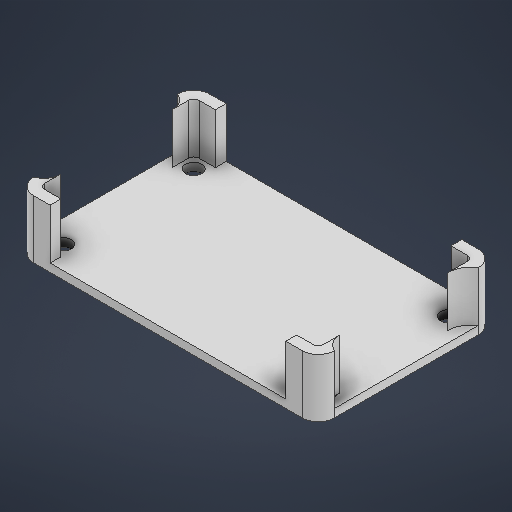
# Autodesk Inventor part: Part4
Saved by Autodesk Inventor 2026.1 (Build 301233020, 233B)
## iProperties
Created: 2025-12-24
Part Number: Part4
Material: Generic
Document SubType Name: Modeling
Designer: ferrm
Density: 1 g/cm^3
Appearance: Default
Author: ferrm
Autodesk Inventor part; units mm, degrees
ref_plane "YZ Plane" through (0, 0, 0) normal (1, 0, 0) x (0, 1, 0)
ref_plane "XZ Plane" through (0, 0, 0) normal (0, 1, 0) x (-1, 0, 0)
ref_plane "XY Plane" through (0, 0, 0) normal (0, 0, 1) x (1, 0, 0)
sketch "Sketch3" plane through (0, 0, 0) normal (0, 1, 0) x (-1, 0, 0)
  line L0 (-25.75, 13.25) -> (-25.75, -13.25)
  line L1 (-24.75, -14.25) -> (24.75, -14.25)
  line L2 (25.75, -13.25) -> (25.75, 13.25)
  line L3 (24.75, 14.25) -> (-24.75, 14.25)
  arc A0 (-25.75, -13.25) -> (-24.75, -14.25) centre (-24.75, -13.25) ccw
  arc A1 (-24.75, 14.25) -> (-25.75, 13.25) centre (-24.75, 13.25) ccw
  arc A2 (25.75, 13.25) -> (24.75, 14.25) centre (24.75, 13.25) ccw
  arc A3 (24.75, -14.25) -> (25.75, -13.25) centre (24.75, -13.25) ccw
  line L4 (24.75, -16.25) -> (-24.75, -16.25)
  arc A4 (-27.75, -13.25) -> (-24.75, -16.25) centre (-24.75, -13.25) ccw
  line L5 (-27.75, -13.25) -> (-27.75, 13.25)
  arc A5 (-24.75, 16.25) -> (-27.75, 13.25) centre (-24.75, 13.25) ccw
  line L6 (-24.75, 16.25) -> (24.75, 16.25)
  arc A6 (27.75, 13.25) -> (24.75, 16.25) centre (24.75, 13.25) ccw
  line L7 (27.75, 13.25) -> (27.75, -13.25)
  arc A7 (24.75, -16.25) -> (27.75, -13.25) centre (24.75, -13.25) ccw
  line L8 (21.75, -16.25) -> (21.75, -14.25)
  line L9 (27.75, -10.25) -> (25.75, -10.25)
  line L10 (25.75, 10.25) -> (27.75, 10.25)
  line L11 (21.75, 14.25) -> (21.75, 16.25)
  line L12 (-21.75, 14.25) -> (-21.75, 16.25)
  line L13 (-25.75, 10.25) -> (-27.75, 10.25)
  line L14 (-25.75, -10.25) -> (-27.75, -10.25)
  line L15 (-21.75, -16.25) -> (-21.75, -14.25)
  line L16 (-21.75, -14.25) -> (-17.75, -14.25)
  arc A8 (-17.75, -14.25) -> (-21.75, -16.25) centre (-15.3911, -23.9678) ccw
  line L17 (-21.75, 14.25) -> (-17.75, 14.25)
  arc A9 (-21.75, 16.25) -> (-17.75, 14.25) centre (-15.3911, 23.9678) ccw
  line L18 (-25.75, -10.25) -> (-25.75, -6.2495)
  line L19 (-25.75, 10.25) -> (-25.75, 6.25)
  arc A10 (-27.75, -10.25) -> (-25.75, -6.2495) centre (-35.468, -3.8913) ccw
  arc A11 (-25.75, 6.25) -> (-27.75, 10.25) centre (-35.4678, 3.8911) ccw
  line L20 (25.75, -10.25) -> (25.75, -6.2495)
  arc A12 (25.75, -6.2495) -> (27.75, -10.25) centre (35.468, -3.8913) ccw
  line L21 (25.75, 10.25) -> (25.75, 6.25)
  arc A13 (27.75, 10.25) -> (25.75, 6.25) centre (35.4678, 3.8911) ccw
  point P0 (0, 0)
  point P1 (0, 0)
  point P2 (-25.75, 14.25)
  point P3 (-25.75, -14.25)
  point P4 (25.75, -14.25)
  point P5 (21.75, 15.25)
  point P6 (-26.75, 10.25)
  dimension "d8" = 28.5
  dimension "d9" = 51.5
  dimension "d10" = 14.25
  dimension "d11" = 25.75
  dimension "d12" = 1
  dimension "d13" = 2
  dimension "d14" = 3
  dimension "d15" = 3
  dimension "d16" = 3
  dimension "d17" = 3
  dimension "d18" = 3
  dimension "d19" = 3
  dimension "d20" = 3
  dimension "d21" = 3
  dimension "d22" = 4
  dimension "d23" = 10
  dimension "d24" = 10
  dimension "d25" = 4
  dimension "d26" = 10
  dimension "d27" = 10
  dimension "d28" = 10
  dimension "d29" = 10
  constraints: 44 end point, 28 point on circle, 28 point on line, 14 centre point, 11 perpendicular, 8 tangent, 3 equal radius, 2 horizontal, 2 midpoint, 1 coincident, 1 vertical, 7 other
  measures "d8" distance of point (-25.75, 14.25) point (-25.75, -14.25)
  measures "d9" distance of point (-25.75, -14.25) point (25.75, -14.25)
  measures "d10" vertical distance of point (0, 0) point (-25.75, -14.25)
  measures "d11" horizontal distance of point (0, 0) point (-25.75, -14.25)
  measures "d12" radius of A0
  measures "d13" distance between parallel lines of L1 L4
  measures "d14" distance of L4.start L8.start
  measures "d15" distance from line of L7.end L9
  measures "d16" distance of L7.start L10.end
  measures "d17" horizontal distance of L6.end point (21.75, 15.25)
  measures "d18" distance of L6.start L12.end
  measures "d19" vertical distance of L5.end point (-26.75, 10.25)
  measures "d20" distance from line of L0.end L14
  measures "d21" distance of L15.start L4.end
  measures "d22" distance of L16.start L16.end
  measures "d23" radius of A8
  measures "d24" radius of A9
  measures "d25" distance of L13.start L19.end
  measures "d26" radius of A10
  measures "d27" radius of A11
  measures "d28" radius of A12
  measures "d29" radius of A13
extrude "Extrusion2" add sketch "Sketch3" along normal blind 3 contours L0 L13 L5 A5 L6 L12 L3 A1 | L0 A11 L13 | L12 A9 L3 | L0 L14 A10 | L14 L0 A0 L1 L15 L4 A4 L5 | L11 L6 A6 L7 L10 L2 A2 L3 | L15 L1 A8 | L8 L1 A3 L2 L9 L7 A7 L4 | L10 A13 L2 | L9 L2 A12
sketch "Sketch4" plane through (0, 0, 0) normal (0, -1, 0) x (1, 0, 0)
  line L0 (-27.75, -13.25) -> (-27.75, -10.25) projected
  arc A0 (-27.75, -13.25) -> (-24.75, -16.25) centre (-24.75, -13.25) ccw projected
  line L1 (-21.75, -16.25) -> (-24.75, -16.25) projected
  line L2 (-24.75, 16.25) -> (-21.75, 16.25) projected
  arc A1 (-24.75, 16.25) -> (-27.75, 13.25) centre (-24.75, 13.25) ccw projected
  line L3 (-27.75, 10.25) -> (-27.75, 13.25) projected
  line L4 (21.75, 16.25) -> (24.75, 16.25) projected
  arc A2 (27.75, 13.25) -> (24.75, 16.25) centre (24.75, 13.25) ccw projected
  line L5 (27.75, 13.25) -> (27.75, 10.25) projected
  line L6 (27.75, -10.25) -> (27.75, -13.25) projected
  arc A3 (24.75, -16.25) -> (27.75, -13.25) centre (24.75, -13.25) ccw projected
  line L7 (24.75, -16.25) -> (21.75, -16.25) projected
  line L8 (-21.75, -16.25) -> (21.75, -16.25)
  line L9 (-27.75, -10.25) -> (-27.75, 10.25)
  line L10 (-25.75, -6.2495) -> (-25.75, -13.25) projected
  line L11 (-21.75, 16.25) -> (-21.75, 14.25) projected
  arc A4 (17.75, 14.25) -> (21.75, 16.25) centre (15.3911, 23.9678) ccw projected
  line L12 (-21.75, 16.25) -> (21.75, 16.25)
  arc A5 (25.75, -6.2495) -> (27.75, -10.25) centre (35.468, -3.8913) ccw projected
  line L13 (27.75, 10.25) -> (27.75, -10.25)
  point P0 (0, 0)
  constraints: 8 end point, 2 horizontal, 1 parallel, 1 vertical
extrude "Extrusion3" add sketch "Sketch4" along normal blind 1.5
sketch "Sketch5" plane through (0, 0, 0) normal (0, 1, 0) x (1, 0, 0)
  line L0 (-21.75, -14.25) -> (-24.75, -14.25) projected
  line L1 (-24.75, -14.25) -> (-24.75, -12.05)
  line L2 (-24.75, -12.05) -> (-23.55, -12.05)
  line L3 (-24.75, 14.25) -> (-21.75, 14.25) projected
  line L4 (-24.75, 14.25) -> (-24.75, 12.05)
  line L5 (-24.75, 12.05) -> (-23.55, 12.05)
  arc A0 (25.75, 13.25) -> (24.75, 14.25) centre (24.75, 13.25) ccw projected
  line L6 (24.75, 14.25) -> (24.75, 12.05)
  line L7 (24.75, 12.05) -> (23.55, 12.05)
  arc A1 (24.75, -14.25) -> (25.75, -13.25) centre (24.75, -13.25) ccw projected
  line L8 (24.75, -14.25) -> (24.75, -12.05)
  line L9 (24.75, -12.05) -> (23.55, -12.05)
  point P0 (0, 0)
  dimension "d34" = 2.2
  dimension "d35" = 1.2
  dimension "d36" = 2.2
  dimension "d37" = 2.2
  dimension "d38" = 1.2
  dimension "d39" = 2.2
  constraints: 16 end point, 4 horizontal, 4 vertical
  measures "d34" distance of L0.end L1.end
  measures "d35" distance of L1.end L2.end
  measures "d36" distance of L3.start L4.end
  measures "d37" distance of L6.start L6.end
  measures "d38" distance of L6.end L7.end
  measures "d39" distance of L8.start L8.end
hole "Hole1" at (-23.55, 0, 12.05) at (-23.55, 0, -12.05) at (23.55, 0, -12.05) at (23.55, 0, 12.05) direction (0, -1, 0) diameter 3 end through all
sketch "Sketch6" plane through (0, 3, 0) normal (0, 1, 0) x (1, 0, 0)
  line L0 (25.75, -6.25) -> (25.75, 6.152)
  line L1 (24.75, -14.25) -> (17.75, -14.25) projected
  line L2 (17.75, -14.25) -> (-21.75, -14.25)
  arc A0 (-25.75, 6.2495) -> (-27.75, 10.25) centre (-35.468, 3.8913) ccw projected
  line L3 (-25.75, -6.25) -> (-25.75, 6.2495)
  line L4 (-24.75, 14.25) -> (-21.75, 14.25) projected
  line L5 (-21.75, 14.25) -> (17.75, 14.25)
  line L6 (25.75, -6.25) -> (25.75, -13.25) projected
  arc A1 (24.75, -16.25) -> (27.75, -13.25) centre (24.75, -13.25) ccw projected
  arc A2 (25.75, -10.25) -> (27.75, -13.25) centre (29, -10.25) ccw
  line L7 (25.75, -6.25) -> (25.75, -13.25) projected
  line L8 (25.75, 13.25) -> (25.75, 6.2495) projected
  arc A3 (27.75, 10.25) -> (25.75, 6.2495) centre (35.468, 3.8913) ccw projected
  line L9 (27.75, 10.25) -> (27.75, 13.25) projected
  line L10 (17.75, 14.25) -> (24.75, 14.25) projected
  arc A4 (17.75, 14.25) -> (21.75, 16.25) centre (15.3911, 23.9678) ccw projected
  line L11 (24.75, 16.25) -> (21.75, 16.25) projected
  line L12 (-27.75, 13.25) -> (-27.75, 10.25) projected
  arc A5 (-25.75, 6.2495) -> (-27.75, 10.25) centre (-35.468, 3.8913) ccw projected
  line L13 (-25.75, 6.2495) -> (-25.75, 13.25) projected
  line L14 (-21.75, 14.25) -> (-21.75, 16.25) projected
  line L15 (-21.75, 16.25) -> (-24.75, 16.25) projected
  arc A6 (-27.75, -10.25) -> (-25.75, -6.25) centre (-35.4678, -3.8911) ccw projected
  line L16 (-25.75, -13.25) -> (-25.75, -6.25) projected
  line L17 (-27.75, -10.25) -> (-27.75, -13.25) projected
  arc A7 (-27.75, -13.25) -> (-24.75, -16.25) centre (-24.75, -13.25) ccw projected
  line L18 (-24.75, -16.25) -> (-21.75, -16.25) projected
  line L19 (-21.75, -16.25) -> (-21.75, -14.25) projected
  arc A8 (21.75, -16.25) -> (17.75, -14.25) centre (15.3911, -23.9678) ccw projected
  line L20 (21.75, -16.25) -> (21.75, -14.25)
  arc A9 (-27.75, -13.25) -> (-25.75, -10.4161) centre (-28.7577, -10.4161) ccw
  arc A10 (27.75, 13.25) -> (25.75, 9.6748) centre (29.9455, 9.6748) ccw
  arc A11 (-25.75, 10.3378) -> (-27.75, 13.25) centre (-28.8703, 10.3378) ccw
  line L21 (21.75, 16.25) -> (21.75, 14.25)
  line L22 (27.75, -13.25) -> (27.75, -10.25) projected
  arc A12 (25.75, -6.25) -> (27.75, -10.25) centre (35.4678, -3.8911) ccw projected
  point P0 (0, 0)
  constraints: 12 end point, 8 point on circle, 6 point on line, 4 centre point, 4 tangent, 2 perpendicular, 2 vertical, 1 horizontal
extrude "Extrusion4" cut sketch "Sketch6" against normal blind 3
sketch "Sketch7" plane through (0, 3, 0) normal (0, 1, 0) x (1, 0, 0)
  arc A0 (25.75, -10.25) -> (27.75, -13.25) centre (29, -10.25) ccw projected
  arc A1 (24.75, -16.25) -> (27.75, -13.25) centre (24.75, -13.25) ccw projected
  arc A2 (24.75, -14.25) -> (25.75, -13.25) centre (24.75, -13.25) ccw projected
  line L0 (25.75, -10.25) -> (25.75, -13.25) projected
  line L1 (24.75, -14.25) -> (21.75, -14.25) projected
  line L2 (21.75, -14.25) -> (21.75, -16.25) projected
  line L3 (21.75, -16.25) -> (24.75, -16.25) projected
  line L4 (-21.75, -14.25) -> (-24.75, -14.25) projected
  line L5 (-21.75, -16.25) -> (-21.75, -14.25) projected
  line L6 (-24.75, -16.25) -> (-21.75, -16.25) projected
  arc A3 (-27.75, -13.25) -> (-24.75, -16.25) centre (-24.75, -13.25) ccw projected
  arc A4 (-27.75, -13.25) -> (-25.75, -10.4161) centre (-28.7577, -10.4161) ccw projected
  line L7 (-25.75, -13.25) -> (-25.75, -10.4161) projected
  arc A5 (-25.75, -13.25) -> (-24.75, -14.25) centre (-24.75, -13.25) ccw projected
  arc A6 (-25.75, 10.3378) -> (-27.75, 13.25) centre (-28.8703, 10.3378) ccw projected
  line L8 (-25.75, 10.3378) -> (-25.75, 13.25) projected
  arc A7 (-24.75, 14.25) -> (-25.75, 13.25) centre (-24.75, 13.25) ccw projected
  line L9 (-24.75, 14.25) -> (-21.75, 14.25) projected
  line L10 (-21.75, 14.25) -> (-21.75, 16.25) projected
  line L11 (-21.75, 16.25) -> (-24.75, 16.25) projected
  arc A8 (-24.75, 16.25) -> (-27.75, 13.25) centre (-24.75, 13.25) ccw projected
  arc A9 (27.75, 13.25) -> (24.75, 16.25) centre (24.75, 13.25) ccw projected
  line L12 (24.75, 16.25) -> (21.75, 16.25) projected
  line L13 (21.75, 16.25) -> (21.75, 14.25) projected
  line L14 (21.75, 14.25) -> (24.75, 14.25) projected
  arc A10 (25.75, 13.25) -> (24.75, 14.25) centre (24.75, 13.25) ccw projected
  line L15 (25.75, 13.25) -> (25.75, 9.6748) projected
  arc A11 (27.75, 13.25) -> (25.75, 9.6748) centre (29.9455, 9.6748) ccw projected
  point P0 (0, 0)
extrude "Extrusion5" add sketch "Sketch7" along normal blind 6.25
body "Solid2"
